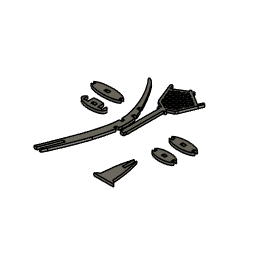
burnathome_model (Autodesk Fusion 360 design; units mm, degrees)
Autodesk Fusion 360 part; units mm, degrees
note: some values were not read from the file. Set by a fixed rule: which sketch regions a step uses.
(part 1 of 2)
sketch "Sketch1" plane through (0, 0, 0) normal (0, 0, 1) x (1, 0, 0)
  spline S0 degree 3 poles (105.7444, 14.5032) (117.4288, 44.6604) (130.3665, 74.6483) (136.8117, 106.4812) knots 0 0 0 0 1 1 1 1
  spline S1 degree 3 poles (135.284, 152.6044) (128.6212, 175.9715) (117.3015, 198.1451) (101.7627, 216.8286) knots 0 0 0 0 1 1 1 1
  spline S2 degree 3 poles (101.7627, 216.8286) (100.2225, 218.6487) (96.6852, 221.8312) (97.531, 222.5321) knots 0 0 0 0 1 1 1 1
  spline S3 degree 3 poles (97.531, 222.5321) (99.4549, 223.9712) (106.4176, 220.3297) (113.8276, 209.9742) knots 0 0 0 0 1 1 1 1
  spline S4 degree 3 poles (113.8276, 209.9742) (127.6672, 190.7251) (139.1986, 169.8205) (148.7703, 148.1491) knots 0 0 0 0 1 1 1 1
  spline S5 degree 3 poles (148.7593, 148.174) (152.834, 138.1049) (152.7256, 126.9178) (152.0453, 116.2604) knots 0 0 0 0 1 1 1 1
  spline S6 degree 3 poles (152.047, 116.2872) (150.3094, 104.2979) (146.4472, 89.1288) (141.1137, 70.5518) knots 0 0 0 0 1 1 1 1
  spline S7 degree 2 poles (161.9789, 170.2352) (154.8849, 179.5494) (137.874, 203.6318) knots 0 0 0 1 1 1
  spline S8 degree 3 poles (137.874, 203.6318) (145.0675, 206.7636) (154.3879, 210.8154) (161.9789, 214.1758) knots 0 0 0 0 1 1 1 1
  spline S9 degree 3 poles (161.9789, 214.1758) (170.0804, 210.3083) (178.4147, 206.771) (186.3736, 202.7014) knots 0 0 0 0 1 1 1 1
  spline S10 degree 3 poles (186.3736, 202.7014) (182.615, 197.9373) (162.2857, 169.7391) (161.9789, 170.2352) knots 0 0 0 0 1 1 1 1
  line L0 (161.9789, 214.1758) -> (161.9789, 165.1) construction
  line L1 (101.7627, 216.8286) -> (100.2225, 218.6487) construction
  line L2 (100.2225, 218.6487) -> (96.6852, 221.8312) construction
  line L3 (96.6852, 221.8312) -> (97.531, 222.5321) construction
  line L4 (97.531, 222.5321) -> (99.4549, 223.9712) construction
  line L5 (99.4549, 223.9712) -> (106.4176, 220.3297) construction
  line L6 (106.4176, 220.3297) -> (113.8276, 209.9742) construction
  line L7 (152.047, 116.2872) -> (150.3094, 104.2979) construction
  line L8 (150.3094, 104.2979) -> (146.4472, 89.1288) construction
  line L9 (146.4472, 89.1288) -> (141.1137, 70.5518) construction
  line L10 (119.1614, 37.5643) -> (123.5466, 35.8761)
  line L11 (123.5466, 35.8761) -> (109.8583, 0.3199)
  line L12 (119.1614, 37.5643) -> (104.7977, 0.254)
  spline S11 degree 3 poles (141.1137, 70.5518) (136.0968, 54.3686) (125.6817, 28.5289) (117.0593, 8.6966) knots 0 0 0 0 0.937383 0.937383 0.937383 0.937383
  line L13 (141.1137, 70.5518) -> (136.0968, 54.3686) construction
  line L14 (136.0968, 54.3686) -> (125.6817, 28.5289) construction
  line L15 (125.6817, 28.5289) -> (117.0593, 8.6966) construction
  spline S12 degree 3 poles (99.568, 0.254) (99.8499, 0.2503) (102.6483, 6.336) (105.7444, 14.5032) knots 0.351989 0.351989 0.351989 0.351989 1 1 1 1
  line L16 (99.568, 0.254) -> (99.8499, 0.2503) construction
  line L17 (99.8499, 0.2503) -> (102.6483, 6.336) construction
  line L18 (102.6483, 6.336) -> (105.7444, 14.5032) construction
  line L19 (202.385, 12.1082) -> (221.4351, 12.1082)
  line L20 (221.4351, 12.1082) -> (221.4351, 36.9579) construction
  line L21 (219.0856, 50.2082) -> (219.0856, 73.0762)
  line L22 (219.0856, 50.2082) -> (221.4351, 50.2082)
  arc A0 (209.8206, 17.9721) -> (202.385, 12.1082) centre (221.435, -4.4018) ccw
  spline S13 degree 5 poles (219.0856, 73.0762) (218.798, 72.0356) (218.2295, 69.9495) (217.3962, 66.8053) (216.327, 62.5819) (215.0787, 57.2456) (213.9414, 51.8447) (212.9362, 46.3723) (212.0737, 40.825) (211.3458, 35.2064) (210.736, 29.5227) (210.3279, 24.9291) (210.0601, 21.4598) (209.8977, 19.1364) (209.8206, 17.9721) knots 0 0 0 0 0 0 0.1 0.2 0.3 0.4 0.5 0.6 0.7 0.8 0.9 1 1 1 1 1 1
  line L23 (240.4851, 12.1082) -> (221.4351, 12.1082)
  arc A1 (240.4851, 12.1082) -> (233.0495, 17.9721) centre (221.4351, -4.4018) ccw
  line L24 (223.7846, 50.2082) -> (223.7846, 73.0762)
  spline S14 degree 5 poles (223.7846, 73.0762) (224.0721, 72.0356) (224.6406, 69.9495) (225.4739, 66.8053) (226.5431, 62.5819) (227.7914, 57.2456) (228.9287, 51.8447) (229.9339, 46.3723) (230.7964, 40.825) (231.5243, 35.2064) (232.1341, 29.5227) (232.5422, 24.9291) (232.81, 21.4598) (232.9724, 19.1364) (233.0495, 17.9721) knots 0 0 0 0 0 0 0.1 0.2 0.3 0.4 0.5 0.6 0.7 0.8 0.9 1 1 1 1 1 1
  line L25 (220.5921, 78.5288) -> (217.579, 67.6235)
  line L26 (210.2086, 23.8294) -> (209.4327, 12.1147)
  line L27 (222.278, 78.5288) -> (225.2911, 67.6235)
  line L28 (232.6616, 23.8294) -> (233.4374, 12.1147)
  line L29 (223.7846, 50.2082) -> (221.4351, 50.2082)
  line L30 (161.9789, 228.6) -> (161.9789, -25.4) construction
  line L31 (139.0297, 126.8561) -> (161.9789, 126.8561) construction
  line L32 (137.237, 162.3529) -> (161.9789, 162.3117) construction
  line L33 (143.7687, 145.0614) -> (161.9789, 145.0614) construction
  line L34 (156.4687, 142.7119) -> (143.7687, 142.7119)
  line L35 (143.7687, 142.7119) -> (143.7687, 147.4109)
  line L36 (143.7687, 147.4109) -> (156.4687, 147.4109)
  line L37 (156.4687, 147.4109) -> (156.4687, 142.7119)
  line L38 (156.4687, 142.7119) -> (143.7687, 147.4109) construction
  line L39 (143.7687, 142.7119) -> (156.4687, 147.4109) construction
  line L40 (161.9789, 108.9422) -> (146.0368, 108.9422) construction
  line L41 (155.5618, 111.2917) -> (146.0368, 111.2917)
  line L42 (146.0368, 111.2917) -> (146.0368, 106.5927)
  line L43 (146.0368, 106.5927) -> (155.5618, 106.5927)
  line L44 (155.5618, 106.5927) -> (155.5618, 111.2917)
  line L45 (155.5618, 111.2917) -> (146.0368, 106.5927) construction
  line L46 (146.0368, 111.2917) -> (155.5618, 106.5927) construction
  line L47 (147.0795, 159.9952) -> (137.237, 159.9952)
  line L48 (137.237, 159.9952) -> (137.237, 164.6942)
  line L49 (137.237, 164.6942) -> (147.0795, 164.6942)
  line L50 (147.0795, 164.6942) -> (147.0795, 159.9952)
  line L51 (147.0795, 159.9952) -> (137.237, 164.6942) construction
  line L52 (137.237, 159.9952) -> (147.0795, 164.6942) construction
  ellipse E0 centre (79.447, 160.9534) end of major axis (109.2158, 160.9534) minor radius 9.525
  line L53 (49.6782, 160.9534) -> (109.2158, 160.9534) construction
  line L54 (79.447, 151.4284) -> (79.447, 170.4784) construction
  line L55 (83.257, 158.6039) -> (75.637, 158.6039)
  line L56 (75.637, 158.6039) -> (75.637, 163.3029)
  line L57 (75.637, 163.3029) -> (83.257, 163.3029)
  line L58 (83.257, 163.3029) -> (83.257, 158.6039)
  line L59 (83.257, 158.6039) -> (75.637, 163.3029) construction
  line L60 (75.637, 158.6039) -> (83.257, 163.3029) construction
  line L61 (132.2063, 162.3613) -> (137.237, 162.3529) construction
  line L62 (137.1951, 145.0614) -> (143.7687, 145.0614) construction
  line L63 (146.0368, 108.9422) -> (137.3129, 108.9422) construction
  line L64 (54.6058, 163.3029) -> (44.7506, 163.3029)
  line L65 (44.7506, 163.3029) -> (44.7506, 158.6039)
  line L66 (44.7506, 158.6039) -> (54.6058, 158.6039)
  line L67 (54.6058, 158.6039) -> (54.6058, 163.3029)
  line L68 (54.6058, 163.3029) -> (44.7506, 158.6039) construction
  line L69 (44.7506, 163.3029) -> (54.6058, 158.6039) construction
  line L70 (104.2882, 158.6039) -> (114.1434, 158.6039)
  line L71 (114.1434, 158.6039) -> (114.1434, 163.3029)
  line L72 (114.1434, 163.3029) -> (104.2882, 163.3029)
  line L73 (104.2882, 163.3029) -> (104.2882, 158.6039)
  line L74 (104.2882, 158.6039) -> (114.1434, 163.3029) construction
  line L75 (114.1434, 158.6039) -> (104.2882, 163.3029) construction
  line L76 (237.743, 142.2845) -> (245.363, 146.9835) construction
  line L77 (259.7902, 146.9835) -> (259.7902, 142.2845)
  line L78 (274.1158, 142.2845) -> (274.1158, 146.9835)
  line L79 (208.9902, 146.9835) -> (223.3158, 142.2845) construction
  line L80 (208.9902, 146.9835) -> (208.9902, 142.2845)
  line L81 (223.3158, 142.2845) -> (223.3158, 146.9835)
  line L82 (259.7902, 142.2845) -> (274.1158, 142.2845)
  line L83 (245.363, 142.2845) -> (237.743, 142.2845)
  line L84 (245.363, 142.2845) -> (237.743, 146.9835) construction
  line L85 (259.7902, 142.2845) -> (274.1158, 146.9835) construction
  line L86 (237.743, 142.2845) -> (237.743, 146.9835)
  line L87 (208.9902, 142.2845) -> (223.3158, 142.2845)
  line L88 (245.363, 146.9835) -> (245.363, 142.2845)
  line L89 (274.1158, 142.2845) -> (259.7902, 146.9835) construction
  line L90 (274.1158, 146.9835) -> (259.7902, 146.9835)
  line L91 (223.3158, 146.9835) -> (208.9902, 146.9835)
  line L92 (237.743, 146.9835) -> (245.363, 146.9835)
  line L93 (223.3158, 146.9835) -> (208.9902, 142.2845) construction
  ellipse E1 centre (241.553, 144.634) end of major axis (266.953, 144.634) minor radius 9.525
  line L94 (216.153, 144.634) -> (266.953, 144.634) construction
  line L95 (241.553, 135.109) -> (241.553, 154.159) construction
  line L96 (91.1889, 125.3656) -> (83.5689, 125.3656)
  line L97 (91.1889, 125.3656) -> (83.5689, 130.0646) construction
  line L98 (83.5689, 130.0646) -> (91.1889, 130.0646)
  line L99 (83.5689, 125.3656) -> (83.5689, 130.0646)
  line L100 (91.1889, 130.0646) -> (91.1889, 125.3656)
  line L101 (83.5689, 125.3656) -> (91.1889, 130.0646) construction
  line L102 (225.1114, 106.1159) -> (225.1114, 110.8149)
  line L103 (268.2914, 106.1159) -> (257.1662, 110.8149) construction
  line L104 (213.9862, 110.8149) -> (225.1114, 106.1159) construction
  line L105 (257.1662, 106.1159) -> (268.2914, 110.8149) construction
  line L106 (244.3138, 106.1159) -> (237.9638, 106.1159)
  line L107 (257.1662, 106.1159) -> (268.2914, 106.1159)
  line L108 (225.1114, 110.8149) -> (213.9862, 110.8149)
  line L109 (244.3138, 106.1159) -> (237.9638, 110.8149) construction
  line L110 (257.1662, 110.8149) -> (257.1662, 106.1159)
  line L111 (213.9862, 110.8149) -> (213.9862, 106.1159)
  line L112 (225.1114, 110.8149) -> (213.9862, 106.1159) construction
  line L113 (213.9862, 106.1159) -> (225.1114, 106.1159)
  line L114 (268.2914, 110.8149) -> (257.1662, 110.8149)
  line L115 (237.9638, 110.8149) -> (244.3138, 110.8149)
  line L116 (237.9638, 106.1159) -> (237.9638, 110.8149)
  line L117 (244.3138, 110.8149) -> (244.3138, 106.1159)
  line L118 (237.9638, 106.1159) -> (244.3138, 110.8149) construction
  ellipse E2 centre (241.1388, 108.4654) end of major axis (262.7288, 108.4654) minor radius 9.525
  line L119 (219.5488, 108.4654) -> (262.7288, 108.4654) construction
  line L120 (241.1388, 98.9404) -> (241.1388, 117.9904) construction
  line L121 (268.2914, 106.1159) -> (268.2914, 110.8149)
  line L122 (158.1689, 176.53) -> (165.7889, 176.53)
  line L123 (165.7889, 176.53) -> (165.7889, 111.4565)
  line L124 (158.1689, 111.4565) -> (158.1689, 176.53)
  spline S15 degree 3 poles (161.8759, 205.8008) (166.2261, 203.7742) (170.5456, 201.8424) (174.7461, 199.881) knots 0.127739 0.127739 0.127739 0.127739 0.652669 0.652669 0.652669 0.652669
  spline S16 degree 3 poles (174.7461, 199.881) (172.3216, 196.5944) (169.4721, 192.7118) (166.7324, 188.9957) (165.1268, 186.8178) (163.5593, 184.6977) (162.1432, 182.7963) knots 0.254809 0.254809 0.254809 0.254809 0.50048 0.50048 0.50048 0.64446 0.64446 0.64446 0.64446
  spline S17 degree 3 poles (162.1432, 182.7963) (159.0509, 187.0323) (155.2878, 192.2652) (150.8627, 198.484) (150.4183, 199.1085) (149.9672, 199.743) (149.5094, 200.3875) knots 0.340954 0.340954 0.340954 0.340954 0.787557 0.787557 0.787557 0.83241 0.83241 0.83241 0.83241
  spline S18 degree 3 poles (149.5094, 200.3875) (153.6089, 202.1746) (157.8877, 204.0444) (161.8759, 205.8008) knots 0.36706 0.36706 0.36706 0.36706 0.864387 0.864387 0.864387 0.864387
  spline S19 degree 3 poles (136.8117, 106.4811) (136.8741, 106.7796) (136.9365, 107.0782) (136.999, 107.3768) (140.1243, 122.3208) (139.7101, 137.9614) (135.2839, 152.6046) knots 0 0 0 0 0.091508 0.091508 0.091508 1.091508 1.091508 1.091508 1.091508
  line L125 (144.1097, 129.2056) -> (133.9497, 129.2056)
  line L126 (133.9497, 129.2056) -> (133.9497, 124.5066)
  line L127 (133.9497, 124.5066) -> (144.1097, 124.5066)
  line L128 (144.1097, 124.5066) -> (144.1097, 129.2056)
  line L129 (144.1097, 129.2056) -> (133.9497, 124.5066) construction
  line L130 (133.9497, 129.2056) -> (144.1097, 124.5066) construction
  line L131 (69.3814, 125.4267) -> (77.7634, 125.4267)
  line L132 (77.7634, 125.4267) -> (77.7634, 136.487)
  line L133 (69.3814, 133.6454) -> (69.3814, 125.4267)
  line L134 (96.7076, 125.4267) -> (105.0896, 125.4267)
  line L135 (105.0896, 125.4267) -> (105.0896, 133.7524)
  line L136 (96.7076, 136.5214) -> (96.7076, 125.4267)
  ellipse E3 centre (87.3789, 127.7151) end of major axis (110.3281, 127.6837) minor radius 9.525 (69.3814, 133.6454) -> (105.0896, 133.7524) ccw
  ellipse E4 centre (87.3789, 127.7151) end of major axis (110.2537, 127.6848) minor radius 9.6559 (96.7076, 136.5214) -> (77.7634, 136.487) ccw
  line L137 (104.7977, 0.254) -> (99.568, 0.254)
  line L138 (158.8039, 111.4565) -> (158.8039, 106.68)
  line L139 (158.8039, 106.68) -> (165.1539, 106.68)
  line L140 (165.1539, 106.68) -> (165.1539, 111.4565)
  line L141 (165.7889, 111.4565) -> (165.1539, 111.4565)
  line L142 (158.8039, 111.4565) -> (158.1689, 111.4565)
  line L143 (109.8583, 0.3199) -> (113.0859, 0.3199)
  line L144 (117.0593, 8.6966) -> (113.0859, 0.3199)
  point P0 (213.0605, 46.8735)
  point P1 (229.8096, 46.8735)
  point P2 (152.4027, 126.8561)
  point P3 (150.1187, 145.0614)
  point P4 (142.1582, 162.3447)
  point P5 (150.7993, 108.9422)
  point P6 (142.1582, 162.3447)
  point P7 (79.447, 160.9534)
  point P8 (49.6782, 160.9534)
  point P9 (109.2158, 160.9534)
  point P10 (241.553, 144.634)
  point P11 (216.153, 144.634)
  point P12 (266.953, 144.634)
  point P13 (87.3789, 127.7151)
  point P14 (64.2667, 127.9032)
  point P15 (110.1696, 127.9032)
  point P16 (241.1388, 108.4654)
  point P17 (219.5488, 108.4654)
  point P18 (262.7288, 108.4654)
  point P19 (161.9789, 176.53)
  point P20 (140.3889, 108.9503)
  point P21 (136.5789, 145.0601)
  point P22 (139.0297, 126.8561)
  point P23 (69.3467, 127.9032)
  dimension "d2" = 4.699
  dimension "d4" = 38.1
  dimension "d6" = 2.3495
  dimension "d9" = 38.1
  dimension "d12" = 12.7
  dimension "d13" = 4.699
  dimension "d16" = 9.525
  dimension "d17" = 4.699
  dimension "d18" = 9.8425
  dimension "d19" = 4.699
  dimension "d20" = 59.5376
  dimension "d21" = 19.05
  dimension "d22" = 7.62
  dimension "d23" = 4.699
  dimension "d24" = 9.8552
  dimension "d25" = 4.699
  dimension "d26" = 9.8552
  dimension "d27" = 4.699
  dimension "d28" = 50.8
  dimension "d29" = 19.05
  dimension "d30" = 7.62
  dimension "d31" = 4.699
  dimension "d32" = 14.3256
  dimension "d33" = 4.699
  dimension "d34" = 14.3256
  dimension "d35" = 4.699
  dimension "d36" = 45.8984
  dimension "d37" = 19.05
  dimension "d38" = 7.62
  dimension "d39" = 4.699
  dimension "d44" = 43.18
  dimension "d45" = 19.05
  dimension "d46" = 6.35
  dimension "d47" = 4.699
  dimension "d48" = 11.1252
  dimension "d49" = 4.699
  dimension "d50" = 11.1252
  dimension "d51" = 4.699
  dimension "d52" = 7.62
  dimension "d54" = 7.62
  dimension "d61" = 21.59
  dimension "d63" = 25.4
  dimension "d64" = 29.7726
  dimension "d65" = 22.9492
  dimension "d66" = 10.16
  dimension "d67" = 4.699
  dimension "d68" = 5.08
  dimension "d70" = 8.382
  dimension "d71" = 8.382
  dimension "d72" = 5.08
  dimension "d74" = 6.35
  constraint vertical L0
  constraint coincident S7.start L0
  constraint perpendicular L10 L12
  constraint perpendicular L10 L11
  constraint horizontal L19
  constraint perpendicular L19 L20
  constraint perpendicular L19 L21
  constraint coincident L20 L22.end
  constraint midpoint L21.end L25
  constraint midpoint A0.start L26
  constraint symmetric L19.start L20 L23.start
  constraint symmetric L19.end L20 L23.end
  constraint symmetric L20 L21.end L24.end
  constraint symmetric L20 L21.start L24.start
  constraint symmetric L20 A0 A1
  constraint symmetric L20 P0 P1
  constraint symmetric L20 A0.start A1.end
  constraint symmetric L20 L22.end L29.end
  constraint symmetric L20 L25.start L27.start
  constraint symmetric L20 L25.end L27.end
  constraint symmetric L20 L26.start L28.start
  constraint symmetric L20 L26.end L28.end
  constraint vertical L30
  constraint coincident L30 L31.end
  constraint perpendicular L30 L31
  constraint coincident S8.end L30
  constraint coincident L0 L32.end
  constraint coincident L30 L33.end
  constraint perpendicular L30 L33
  constraint coincident L31 P2
  constraint coincident S5 P2
  constraint horizontal L34
  constraint perpendicular L34 L35
  constraint parallel L34 L36
  constraint parallel L35 L37
  constraint coincident L38 P3
  constraint coincident L39 P3
  constraint coincident L33 P3
  constraint coincident S4 P3
  constraint coincident L32 P6
  constraint coincident S4 P6
  constraint coincident L30 L40.start
  constraint perpendicular L30 L40
  constraint horizontal L41
  constraint perpendicular L41 L42
  constraint parallel L41 L43
  constraint parallel L42 L44
  constraint coincident L45 P5
  constraint coincident L46 P5
  constraint coincident S6 P5
  constraint coincident L40 P5
  constraint horizontal L47
  constraint perpendicular L47 L48
  constraint parallel L47 L49
  constraint parallel L48 L50
  constraint coincident L51 P6
  constraint coincident L52 P6
  constraint coincident P6 P4
  constraint coincident S1 L61.start
  constraint coincident L62.start S19
  constraint coincident L63.end S19
  constraint horizontal L53
  constraint coincident E0 P8
  constraint coincident E0 P9
  constraint coincident E0 L54.start
  constraint coincident E0 L54.end
  constraint horizontal L55
  constraint perpendicular L55 L56
  constraint parallel L55 L57
  constraint parallel L56 L58
  constraint coincident L59 P7
  constraint coincident L60 P7
  constraint coincident P7 E0.centre
  constraint coincident L48 L32.start
  constraint coincident P6 L61
  constraint coincident L35 L33.start
  constraint perpendicular L30 L62
  constraint coincident L42 L40.end
  constraint perpendicular L30 L63
  constraint horizontal L64
  constraint perpendicular L64 L65
  constraint parallel L64 L66
  constraint parallel L65 L67
  constraint coincident L68 P8
  constraint coincident L69 P8
  constraint coincident P8 L53.start
  constraint horizontal L70
  constraint perpendicular L70 L71
  constraint parallel L70 L72
  constraint parallel L71 L73
  constraint coincident L74 P9
  constraint coincident L75 P9
  constraint coincident P9 L53.end
  constraint horizontal L94
  constraint coincident P11 E1
  constraint coincident P12 E1
  constraint coincident L95.start E1
  constraint coincident L95.end E1
  constraint horizontal L83
  constraint perpendicular L83 L86
  constraint parallel L83 L92
  constraint parallel L86 L88
  constraint coincident P10 L84
  constraint coincident P10 L76
  constraint coincident P10 E1.centre
  constraint horizontal L91
  constraint perpendicular L80 L91
  constraint parallel L87 L91
  constraint parallel L80 L81
  constraint coincident P11 L93
  constraint coincident P11 L79
  constraint coincident P11 L94.start
  constraint horizontal L82
  constraint perpendicular L78 L82
  constraint parallel L82 L90
  constraint parallel L77 L78
  constraint coincident P12 L85
  constraint coincident P12 L89
  constraint coincident P12 L94.end
  constraint horizontal L96
  constraint perpendicular L96 L99
  constraint parallel L96 L98
  constraint parallel L99 L100
  constraint coincident P13 L97
  constraint coincident P13 L101
  constraint coincident P13 E3.centre
  constraint horizontal L119
  constraint coincident P17 E2
  constraint coincident P18 E2
  constraint coincident L120.start E2
  constraint coincident L120.end E2
  constraint horizontal L106
  constraint perpendicular L106 L116
  constraint parallel L106 L115
  constraint parallel L116 L117
  constraint coincident P16 L109
  constraint coincident P16 L118
  constraint coincident P16 E2.centre
  constraint horizontal L108
  constraint perpendicular L108 L111
  constraint parallel L108 L113
  constraint parallel L102 L111
  constraint coincident P17 L112
  constraint coincident P17 L104
  constraint coincident P17 L119.start
  constraint horizontal L107
  constraint perpendicular L107 L121
  constraint parallel L107 L114
  constraint parallel L110 L121
  constraint coincident P18 L105
  constraint coincident P18 L103
  constraint coincident P18 L119.end
  constraint horizontal L122
  constraint vertical L123
  constraint horizontal L141
  constraint vertical L124
  constraint midpoint L122 P19
  constraint coincident L30 P19
  constraint coincident S19 P22
  constraint horizontal L125
  constraint perpendicular L125 L126
  constraint parallel L125 L127
  constraint parallel L126 L128
  constraint coincident L129 P22
  constraint coincident L130 P22
  constraint coincident P22 L31.start
  constraint horizontal L131
  constraint vertical L132
  constraint vertical L133
  constraint horizontal L134
  constraint vertical L135
  constraint vertical L136
  constraint concentric E3 E4
  constraint horizontal L137
  constraint coincident S12.start L16.start
  constraint coincident L138.start L141
  constraint perpendicular L138 L141
  constraint perpendicular L138 L139
  constraint perpendicular L140 L141
  constraint collinear L141 L142
  constraint equal L141 L142
  constraint horizontal L143
  measures "d2" distance of L10.start L10.end
  measures "d4" distance of L10.end L11.end
  measures "d6" distance of L20 L21
  measures "d9" distance of L19 L22
  measures "d12" distance of L35.end L36.end
  measures "d13" distance of L34.end L35.end
  measures "d16" distance of L42.end L43.end
  measures "d17" distance of L41.end L42.end
  measures "d18" distance of L48.end L49.end
  measures "d19" distance of L47.end L48.end
  measures "d20" distance of E0
  measures "d22" distance of L56.end L57.end
  measures "d23" distance of L55.end L56.end
  measures "d24" distance of L65.end L66.end
  measures "d25" distance of L64.end L65.end
  measures "d26" distance of L71.end L72.end
  measures "d27" distance of L70.end L71.end
  measures "d28" distance of E1
  measures "d30" distance of L84.end L76.end
  measures "d31" distance of L84.end L76.start
  measures "d32" distance of L79.end L80.end
  measures "d33" distance of L79.start L80.end
  measures "d34" distance of L78.end L77.start
  measures "d35" distance of L78.start L78.end
  measures "d36" distance of E3
  measures "d38" distance of L97.end L98.end
  measures "d39" distance of L97.end L96.end
  measures "d44" distance of E2
  measures "d46" distance of L109.end L115.end
  measures "d47" distance of L109.end L106.end
  measures "d48" distance of L102.start L111.end
  measures "d49" distance of L104.start L111.end
  measures "d50" distance of L105.end L103.end
  measures "d51" distance of L103.start L105.end
  measures "d52" distance of L122.start L122.end
  measures "d61" distance of L40.start P20
  measures "d63" distance of L33.end P21
  measures "d64" horizontal distance of L32.end L61.start
  measures "d65" distance of L31.end P22
  measures "d66" distance of L126.end L127.end
  measures "d67" distance of L125.end L126.end
  measures "d68" distance of P14 P23
  measures "d70" distance of L131.start L131.end
  measures "d71" distance of L134.start L134.end
  measures "d72" distance of P15 L135
  measures "d74" distance of L138.end L139.end
extrude "Extrude2" add sketch "Sketch1" along normal blind 4.699 contours S0 S1 S2 S3 S4 S5 S6 L10 L11 L12 S11 S12 L34 L35 L36 L41 L42 L43 L47 L48 L49 S19 L125 L127 L128 L137 L143 L144 | S7 S10 L123 L124 L138 L139 L140 L141 L142 | S7 S10 L122 L123 L124 | S7 S8 S9 S10 L122 L123 L124 | L19 L21 L22 A0 S13 L23 A1 L24 S14 L29 | E0 L64 L66 L67 L70 L72 L73 | L77 L81 L82 L87 L90 L91 E1 | L102 L107 L108 L110 L113 L114 E2 | L131 L132 L133 L134 L135 L136 E3 E4 makes body 1 at (252.4331, 149.0861, 0) makes body 2 at (79.6986, 130.6594, 0) makes body 3 at (175.6362, 192.5122, 0) makes body 4 at (251.5125, 112.6791, 0) makes body 5 at (70.1789, 161.7848, 0) makes body 6 at (221.4351, 26.658, 0) makes body 7 at (133.7227, 78.9656, 0)
sketch "Sketch2" plane through (0, 0, 4.699) normal (0, 0, 1) x (-1, 0, 0)
  line L0 (-158.8039, -106.68) -> (-165.1539, -106.68)
  line L1 (-165.1539, -106.68) -> (-165.1539, -111.4565)
  line L2 (-165.1539, -111.4565) -> (-165.7889, -111.4565)
  line L3 (-165.7889, -111.4565) -> (-165.7889, -174.9541)
  line L4 (-158.1689, -175.331) -> (-158.1689, -111.4565)
  line L5 (-158.1689, -111.4565) -> (-158.8039, -111.4565)
  line L6 (-158.8039, -111.4565) -> (-158.8039, -106.68)
  line L7 (-168.7102, -180.8892) -> (-170.2391, -183.9833)
  line L8 (-191.2572, -223.0614) -> (-194.8572, -232.3981)
  line L9 (-191.7134, -233.6497) -> (-188.2271, -224.8966)
  line L10 (-134.3845, -219.435) -> (-143.8837, -195.7123)
  line L11 (-165.9602, -186.0971) -> (-178.2439, -192.1658)
  line L12 (-188.2271, -224.8966) -> (-165.345, -239.08)
  line L13 (-165.2823, -243.1079) -> (-162.0641, -241.1134)
  line L14 (-157.0243, -240.1702) -> (-158.7831, -239.08)
  line L15 (-153.8892, -183.9833) -> (-155.4181, -180.8892)
  line L16 (-129.2709, -232.3981) -> (-132.8709, -223.0612)
  line L17 (-170.2391, -183.9833) -> (-165.9602, -186.0971)
  line L18 (-162.0641, -241.1134) -> (-158.8458, -243.1079)
  line L19 (-194.8572, -232.3981) -> (-191.7134, -233.6497)
  line L20 (-145.8842, -192.1658) -> (-158.1682, -186.0971)
  line L21 (-135.9013, -224.8966) -> (-132.4147, -233.6497)
  line L22 (-165.345, -239.08) -> (-167.1041, -240.1702)
  line L23 (-165.7889, -182.3323) -> (-168.7102, -180.8892)
  line L24 (-180.2447, -195.7123) -> (-189.7436, -219.435)
  line L25 (-132.4147, -233.6497) -> (-129.2709, -232.3981)
  line L26 (-155.4181, -180.8892) -> (-158.1689, -182.2481)
  line L27 (-158.8458, -243.1079) -> (-157.0243, -240.1702)
  line L28 (-158.1682, -186.0971) -> (-153.8892, -183.9833)
  line L29 (-158.7831, -239.08) -> (-135.9013, -224.8966)
  line L30 (-167.1041, -240.1702) -> (-165.2823, -243.1079)
  line L31 (-150.8628, -193.556) -> (-150.8628, -195.1061)
  line L32 (-150.8628, -195.1061) -> (-147.768, -195.1061)
  line L33 (-147.768, -195.1061) -> (-147.7791, -195.0794)
  line L34 (-147.7791, -195.0794) -> (-150.8628, -193.556)
  line L35 (-152.1466, -192.9219) -> (-157.4944, -190.2798)
  line L36 (-152.1466, -195.1061) -> (-152.1466, -192.9219)
  line L37 (-157.4944, -190.2798) -> (-157.4944, -195.1061)
  line L38 (-157.4944, -195.1061) -> (-152.1466, -195.1061)
  line L39 (-161.8363, -188.1347) -> (-164.116, -189.2274)
  line L40 (-164.116, -195.1061) -> (-158.7509, -195.1061)
  line L41 (-158.7509, -189.6587) -> (-161.8363, -188.1347)
  line L42 (-164.116, -189.2274) -> (-164.116, -195.1061)
  line L43 (-158.7509, -195.1061) -> (-158.7509, -189.6587)
  line L44 (-165.3649, -195.1061) -> (-165.3649, -189.8259)
  line L45 (-170.8485, -192.4544) -> (-170.8485, -195.1061)
  line L46 (-170.8485, -195.1061) -> (-165.3649, -195.1061)
  line L47 (-165.3649, -189.8259) -> (-170.8485, -192.4544)
  line L48 (-172.1153, -195.1061) -> (-172.1153, -193.0618)
  line L49 (-176.3048, -195.07) -> (-176.3191, -195.1061)
  line L50 (-172.1153, -193.0618) -> (-176.3048, -195.07)
  line L51 (-176.3191, -195.1061) -> (-172.1153, -195.1061)
  line L52 (-145.6673, -201.6101) -> (-145.6673, -200.3815)
  line L53 (-150.8628, -196.4098) -> (-150.8628, -201.6101)
  line L54 (-150.8628, -201.6101) -> (-145.6673, -201.6101)
  line L55 (-145.6673, -200.3815) -> (-147.2493, -196.4098)
  line L56 (-147.2493, -196.4098) -> (-150.8628, -196.4098)
  line L57 (-152.1466, -196.4098) -> (-157.4944, -196.4098)
  line L58 (-157.4944, -201.6101) -> (-152.1466, -201.6101)
  line L59 (-157.4944, -196.4098) -> (-157.4944, -201.6101)
  line L60 (-152.1466, -201.6101) -> (-152.1466, -196.4098)
  line L61 (-158.7509, -201.6101) -> (-158.7509, -196.4098)
  line L62 (-158.7509, -196.4098) -> (-164.116, -196.4098)
  line L63 (-164.116, -201.6101) -> (-158.7509, -201.6101)
  line L64 (-164.116, -196.4098) -> (-164.116, -201.6101)
  line L65 (-165.3649, -201.6101) -> (-165.3649, -196.4098)
  line L66 (-170.8485, -196.4098) -> (-170.8485, -201.6101)
  line L67 (-165.3649, -196.4098) -> (-170.8485, -196.4098)
  line L68 (-170.8485, -201.6101) -> (-165.3649, -201.6101)
  line L69 (-172.1153, -196.4098) -> (-176.8407, -196.4098)
  line L70 (-178.9203, -201.6101) -> (-172.1153, -201.6101)
  line L71 (-176.8407, -196.4098) -> (-178.9203, -201.6101)
  line L72 (-172.1153, -201.6101) -> (-172.1153, -196.4098)
  line L73 (-142.5384, -208.2364) -> (-144.3532, -203.6796)
  line L74 (-144.3532, -208.2364) -> (-142.5384, -208.2364)
  line L75 (-144.3532, -203.6796) -> (-144.3532, -208.2364)
  line L76 (-150.8628, -202.894) -> (-150.8628, -208.2364)
  line L77 (-145.6673, -202.894) -> (-150.8628, -202.894)
  line L78 (-150.8628, -208.2364) -> (-145.6673, -208.2364)
  line L79 (-145.6673, -208.2364) -> (-145.6673, -202.894)
  line L80 (-152.1466, -202.894) -> (-157.4944, -202.894)
  line L81 (-157.4944, -202.894) -> (-157.4944, -208.2364)
  line L82 (-157.4944, -208.2364) -> (-152.1466, -208.2364)
  line L83 (-152.1466, -208.2364) -> (-152.1466, -202.894)
  line L84 (-158.7509, -208.2364) -> (-158.7509, -202.894)
  line L85 (-164.116, -208.2364) -> (-158.7509, -208.2364)
  line L86 (-158.7509, -202.894) -> (-164.116, -202.894)
  line L87 (-164.116, -202.894) -> (-164.116, -208.2364)
  line L88 (-170.8485, -208.2364) -> (-165.3649, -208.2364)
  line L89 (-165.3649, -208.2364) -> (-165.3649, -202.894)
  line L90 (-170.8485, -202.894) -> (-170.8485, -208.2364)
  line L91 (-165.3649, -202.894) -> (-170.8485, -202.894)
  line L92 (-179.175, -208.2364) -> (-172.1153, -208.2364)
  line L93 (-172.1153, -208.2364) -> (-172.1153, -202.894)
  line L94 (-172.1153, -202.894) -> (-179.175, -202.894)
  line L95 (-179.175, -202.894) -> (-179.175, -208.2364)
  line L96 (-181.031, -208.2364) -> (-180.9883, -208.2364)
  line L97 (-142.0333, -209.5039) -> (-144.3532, -209.5039)
  line L98 (-139.8995, -214.8606) -> (-142.0333, -209.5039)
  line L99 (-144.3532, -209.5039) -> (-144.3532, -214.8606)
  line L100 (-144.3532, -214.8606) -> (-139.8995, -214.8606)
  line L101 (-145.6673, -214.8606) -> (-145.6673, -209.5039)
  line L102 (-145.6673, -209.5039) -> (-150.8628, -209.5039)
  line L103 (-150.8628, -209.5039) -> (-150.8628, -214.8606)
  line L104 (-150.8628, -214.8606) -> (-145.6673, -214.8606)
  line L105 (-157.4944, -209.5039) -> (-157.4944, -214.8606)
  line L106 (-157.4944, -214.8606) -> (-152.1466, -214.8606)
  line L107 (-152.1466, -209.5039) -> (-157.4944, -209.5039)
  line L108 (-152.1466, -214.8606) -> (-152.1466, -209.5039)
  line L109 (-164.116, -209.5039) -> (-164.116, -214.8606)
  line L110 (-164.116, -214.8606) -> (-158.7509, -214.8606)
  line L111 (-158.7509, -214.8606) -> (-158.7509, -209.5039)
  line L112 (-158.7509, -209.5039) -> (-164.116, -209.5039)
  line L113 (-165.3649, -209.5039) -> (-170.8485, -209.5039)
  line L114 (-170.8485, -209.5039) -> (-170.8485, -214.8606)
  line L115 (-165.3649, -214.8606) -> (-165.3649, -209.5039)
  line L116 (-170.8485, -214.8606) -> (-165.3649, -214.8606)
  line L117 (-172.1153, -209.5039) -> (-179.175, -209.5039)
  line L118 (-172.1153, -214.8606) -> (-172.1153, -209.5039)
  line L119 (-179.175, -209.5039) -> (-179.175, -214.8606)
  line L120 (-179.175, -214.8606) -> (-172.1153, -214.8606)
  line L121 (-180.4883, -214.8606) -> (-180.4883, -209.5039)
  line L122 (-184.2184, -214.8606) -> (-180.4883, -214.8606)
  line L123 (-182.0764, -209.5039) -> (-184.2184, -214.8606)
  line L124 (-180.4883, -209.5039) -> (-182.0764, -209.5039)
  line L125 (-137.2111, -221.6104) -> (-139.4, -216.1156)
  line L126 (-139.4, -216.1156) -> (-144.3532, -216.1156)
  line L127 (-144.3532, -221.6104) -> (-137.2111, -221.6104)
  line L128 (-144.3532, -216.1156) -> (-144.3532, -221.6104)
  line L129 (-145.6673, -216.1156) -> (-150.8628, -216.1156)
  line L130 (-150.8628, -216.1156) -> (-150.8628, -221.6104)
  line L131 (-145.6673, -221.6104) -> (-145.6673, -216.1156)
  line L132 (-150.8628, -221.6104) -> (-145.6673, -221.6104)
  line L133 (-152.1466, -221.6104) -> (-152.1466, -216.1156)
  line L134 (-157.4944, -221.6104) -> (-152.1466, -221.6104)
  line L135 (-157.4944, -216.1156) -> (-157.4944, -221.6104)
  line L136 (-152.1466, -216.1156) -> (-157.4944, -216.1156)
  line L137 (-158.7509, -221.6104) -> (-158.7509, -216.1156)
  line L138 (-164.116, -221.6104) -> (-158.7509, -221.6104)
  line L139 (-158.7509, -216.1156) -> (-164.116, -216.1156)
  line L140 (-164.116, -216.1156) -> (-164.116, -221.6104)
  line L141 (-165.3649, -216.1156) -> (-170.8485, -216.1156)
  line L142 (-170.8485, -216.1156) -> (-170.8485, -221.6104)
  line L143 (-165.3649, -221.6104) -> (-165.3649, -216.1156)
  line L144 (-170.8485, -221.6104) -> (-165.3649, -221.6104)
  line L145 (-179.175, -216.1156) -> (-179.175, -221.6104)
  line L146 (-172.1153, -216.1156) -> (-179.175, -216.1156)
  line L147 (-179.175, -221.6104) -> (-172.1153, -221.6104)
  line L148 (-172.1153, -221.6104) -> (-172.1153, -216.1156)
  line L149 (-180.4883, -221.6104) -> (-180.4883, -216.1156)
  line L150 (-180.4883, -216.1156) -> (-184.7207, -216.1156)
  line L151 (-184.7207, -216.1156) -> (-186.9179, -221.6104)
  line L152 (-186.9179, -221.6104) -> (-180.4883, -221.6104)
  line L153 (-184.9329, -222.8483) -> (-180.4883, -225.5534)
  line L154 (-180.4883, -225.5534) -> (-180.4883, -222.8483)
  line L155 (-180.4883, -222.8483) -> (-184.9329, -222.8483)
  line L156 (-144.3532, -222.8483) -> (-144.3532, -226.0681)
  line L157 (-144.3532, -226.0681) -> (-139.1589, -222.8483)
  line L158 (-139.1589, -222.8483) -> (-144.3532, -222.8483)
  line L159 (-145.6673, -226.8822) -> (-145.6673, -222.8483)
  line L160 (-150.8628, -229.9223) -> (-150.5712, -229.9223)
  line L161 (-145.6673, -222.8483) -> (-150.8628, -222.8483)
  line L162 (-150.5712, -229.9223) -> (-145.6673, -226.8822)
  line L163 (-150.8628, -222.8483) -> (-150.8628, -229.9223)
  line L164 (-157.4944, -222.8483) -> (-157.4944, -229.9223)
  line L165 (-152.1466, -229.9223) -> (-152.1466, -222.8483)
  line L166 (-157.4944, -229.9223) -> (-152.1466, -229.9223)
  line L167 (-152.1466, -222.8483) -> (-157.4944, -222.8483)
  line L168 (-158.7509, -222.8483) -> (-164.116, -222.8483)
  line L169 (-164.116, -229.9223) -> (-158.7509, -229.9223)
  line L170 (-158.7509, -229.9223) -> (-158.7509, -222.8483)
  line L171 (-164.116, -222.8483) -> (-164.116, -229.9223)
  line L172 (-170.8485, -222.8483) -> (-170.8485, -229.9223)
  line L173 (-165.3649, -229.9223) -> (-165.3649, -222.8483)
  line L174 (-165.3649, -222.8483) -> (-170.8485, -222.8483)
  line L175 (-170.8485, -229.9223) -> (-165.3649, -229.9223)
  line L176 (-179.175, -226.3526) -> (-173.31, -229.9223)
  line L177 (-172.1153, -222.8483) -> (-179.175, -222.8483)
  line L178 (-173.31, -229.9223) -> (-172.1153, -229.9223)
  line L179 (-179.175, -222.8483) -> (-179.175, -226.3526)
  line L180 (-172.1153, -229.9223) -> (-172.1153, -222.8483)
  line L181 (-157.4944, -231.2356) -> (-157.4944, -234.2135)
  line L182 (-152.6899, -231.2356) -> (-157.4944, -231.2356)
  line L183 (-157.4944, -234.2135) -> (-152.6899, -231.2356)
  line L184 (-165.3649, -234.7576) -> (-165.3649, -231.2356)
  line L185 (-165.3649, -231.2356) -> (-170.8485, -231.2356)
  line L186 (-170.8485, -231.2356) -> (-170.8485, -231.4199)
  line L187 (-170.8485, -231.4199) -> (-165.3649, -234.7576)
  line L188 (-161.637, -236.7813) -> (-158.947, -235.114)
  line L189 (-163.8746, -231.4856) -> (-163.8746, -235.4192)
  line L190 (-158.947, -231.4856) -> (-163.8746, -231.4856)
  line L191 (-163.8746, -235.4192) -> (-161.637, -236.7813)
  line L192 (-158.947, -235.114) -> (-158.947, -231.4856)
  line L193 (-191.2572, -223.0614) -> (-180.2447, -195.7123)
  line L194 (-178.2439, -192.1658) -> (-180.2447, -195.7123)
  line L195 (-145.8842, -192.1658) -> (-143.8837, -195.7123)
  line L196 (-134.3845, -219.435) -> (-132.8709, -223.0612)
  line L197 (-158.1689, -175.331) -> (-158.1689, -182.2481)
  line L198 (-165.7889, -174.9541) -> (-165.7889, -182.3323)
  line L199 (-163.3746, -235.1382) -> (-161.6393, -236.1945)
  line L200 (-161.6393, -236.1945) -> (-159.447, -234.8356)
  line L201 (-159.447, -234.8356) -> (-159.447, -231.9856)
  line L202 (-159.447, -231.9856) -> (-163.3746, -231.9856)
  line L203 (-163.3746, -231.9856) -> (-163.3746, -235.1382)
  line L204 (-169.3681, -231.7356) -> (-165.8649, -233.8679)
  line L205 (-165.8649, -233.8679) -> (-165.8649, -231.7356)
  line L206 (-165.8649, -231.7356) -> (-169.3681, -231.7356)
  line L207 (-156.9944, -233.3153) -> (-154.4457, -231.7356)
  line L208 (-154.4457, -231.7356) -> (-156.9944, -231.7356)
  line L209 (-156.9944, -231.7356) -> (-156.9944, -233.3153)
  line L210 (-173.1698, -229.4223) -> (-172.6153, -229.4223)
  line L211 (-172.6153, -229.4223) -> (-172.6153, -223.3483)
  line L212 (-172.6153, -223.3483) -> (-178.675, -223.3483)
  line L213 (-178.675, -223.3483) -> (-178.675, -226.0716)
  line L214 (-178.675, -226.0716) -> (-173.1698, -229.4223)
  line L215 (-180.9883, -223.3483) -> (-183.1496, -223.3483)
  line L216 (-183.1496, -223.3483) -> (-180.9883, -224.6638)
  line L217 (-180.9883, -224.6638) -> (-180.9883, -223.3483)
  line L218 (-170.3485, -229.4223) -> (-165.8649, -229.4223)
  line L219 (-165.8649, -229.4223) -> (-165.8649, -223.3483)
  line L220 (-165.8649, -223.3483) -> (-170.3485, -223.3483)
  line L221 (-170.3485, -223.3483) -> (-170.3485, -229.4223)
  line L222 (-163.616, -229.4223) -> (-159.2509, -229.4223)
  line L223 (-159.2509, -229.4223) -> (-159.2509, -223.3483)
  line L224 (-159.2509, -223.3483) -> (-163.616, -223.3483)
  line L225 (-163.616, -223.3483) -> (-163.616, -229.4223)
  line L226 (-156.9944, -229.4223) -> (-152.6466, -229.4223)
  line L227 (-152.6466, -229.4223) -> (-152.6466, -223.3483)
  line L228 (-152.6466, -223.3483) -> (-156.9944, -223.3483)
  line L229 (-156.9944, -223.3483) -> (-156.9944, -229.4223)
  line L230 (-150.3628, -223.3483) -> (-150.3628, -229.2048)
  line L231 (-150.3628, -229.2048) -> (-146.1673, -226.6039)
  line L232 (-146.1673, -226.6039) -> (-146.1673, -223.3483)
  line L233 (-146.1673, -223.3483) -> (-150.3628, -223.3483)
  line L234 (-143.8532, -223.3483) -> (-143.8532, -225.1699)
  line L235 (-143.8532, -225.1699) -> (-140.9146, -223.3483)
  line L236 (-140.9146, -223.3483) -> (-143.8532, -223.3483)
  line L237 (-184.3821, -216.6156) -> (-186.1794, -221.1104)
  line L238 (-186.1794, -221.1104) -> (-180.9883, -221.1104)
  line L239 (-180.9883, -221.1104) -> (-180.9883, -216.6156)
  line L240 (-180.9883, -216.6156) -> (-184.3821, -216.6156)
  line L241 (-178.675, -216.6156) -> (-178.675, -221.1104)
  line L242 (-178.675, -221.1104) -> (-172.6153, -221.1104)
  line L243 (-172.6153, -221.1104) -> (-172.6153, -216.6156)
  line L244 (-172.6153, -216.6156) -> (-178.675, -216.6156)
  line L245 (-143.8532, -221.1104) -> (-137.9485, -221.1104)
  line L246 (-137.9485, -221.1104) -> (-139.739, -216.6156)
  line L247 (-139.739, -216.6156) -> (-143.8532, -216.6156)
  line L248 (-143.8532, -216.6156) -> (-143.8532, -221.1104)
  line L249 (-170.3485, -221.1104) -> (-165.8649, -221.1104)
  line L250 (-165.8649, -221.1104) -> (-165.8649, -216.6156)
  line L251 (-165.8649, -216.6156) -> (-170.3485, -216.6156)
  line L252 (-170.3485, -216.6156) -> (-170.3485, -221.1104)
  line L253 (-146.1673, -221.1104) -> (-146.1673, -216.6156)
  line L254 (-146.1673, -216.6156) -> (-150.3628, -216.6156)
  line L255 (-150.3628, -216.6156) -> (-150.3628, -221.1104)
  line L256 (-150.3628, -221.1104) -> (-146.1673, -221.1104)
  line L257 (-156.9944, -216.6156) -> (-156.9944, -221.1104)
  line L258 (-156.9944, -221.1104) -> (-152.6466, -221.1104)
  line L259 (-152.6466, -221.1104) -> (-152.6466, -216.6156)
  line L260 (-152.6466, -216.6156) -> (-156.9944, -216.6156)
  line L261 (-163.616, -216.6156) -> (-163.616, -221.1104)
  line L262 (-163.616, -221.1104) -> (-159.2509, -221.1104)
  line L263 (-159.2509, -221.1104) -> (-159.2509, -216.6156)
  line L264 (-159.2509, -216.6156) -> (-163.616, -216.6156)
  line L265 (-180.9883, -210.0039) -> (-181.7379, -210.0039)
  line L266 (-181.7379, -210.0039) -> (-183.4799, -214.3606)
  line L267 (-183.4799, -214.3606) -> (-180.9883, -214.3606)
  line L268 (-180.9883, -214.3606) -> (-180.9883, -210.0039)
  line L269 (-142.3724, -210.0039) -> (-143.8532, -210.0039)
  line L270 (-143.8532, -210.0039) -> (-143.8532, -214.3606)
  line L271 (-143.8532, -214.3606) -> (-140.6369, -214.3606)
  line L272 (-140.6369, -214.3606) -> (-142.3724, -210.0039)
  line L273 (-163.616, -214.3606) -> (-159.2509, -214.3606)
  line L274 (-159.2509, -214.3606) -> (-159.2509, -210.0039)
  line L275 (-159.2509, -210.0039) -> (-163.616, -210.0039)
  line L276 (-163.616, -210.0039) -> (-163.616, -214.3606)
  line L277 (-152.6466, -210.0039) -> (-156.9944, -210.0039)
  line L278 (-156.9944, -210.0039) -> (-156.9944, -214.3606)
  line L279 (-156.9944, -214.3606) -> (-152.6466, -214.3606)
  line L280 (-152.6466, -214.3606) -> (-152.6466, -210.0039)
  line L281 (-146.1673, -210.0039) -> (-150.3628, -210.0039)
  line L282 (-150.3628, -210.0039) -> (-150.3628, -214.3606)
  line L283 (-150.3628, -214.3606) -> (-146.1673, -214.3606)
  line L284 (-146.1673, -214.3606) -> (-146.1673, -210.0039)
  line L285 (-170.3485, -210.0039) -> (-170.3485, -214.3606)
  line L286 (-170.3485, -214.3606) -> (-165.8649, -214.3606)
  line L287 (-165.8649, -214.3606) -> (-165.8649, -210.0039)
  line L288 (-165.8649, -210.0039) -> (-170.3485, -210.0039)
  line L289 (-172.6153, -210.0039) -> (-178.675, -210.0039)
  line L290 (-178.675, -210.0039) -> (-178.675, -214.3606)
  line L291 (-178.675, -214.3606) -> (-172.6153, -214.3606)
  line L292 (-172.6153, -214.3606) -> (-172.6153, -210.0039)
  line L293 (-143.2758, -207.7364) -> (-143.8532, -206.2865)
  line L294 (-143.8532, -206.2865) -> (-143.8532, -207.7364)
  line L295 (-143.8532, -207.7364) -> (-143.2758, -207.7364)
  line L296 (-146.1673, -207.7364) -> (-146.1673, -203.394)
  line L297 (-146.1673, -203.394) -> (-150.3628, -203.394)
  line L298 (-150.3628, -203.394) -> (-150.3628, -207.7364)
  line L299 (-150.3628, -207.7364) -> (-146.1673, -207.7364)
  line L300 (-152.6466, -207.7364) -> (-152.6466, -203.394)
  line L301 (-152.6466, -203.394) -> (-156.9944, -203.394)
  line L302 (-156.9944, -203.394) -> (-156.9944, -207.7364)
  line L303 (-156.9944, -207.7364) -> (-152.6466, -207.7364)
  line L304 (-159.2509, -207.7364) -> (-159.2509, -203.394)
  line L305 (-159.2509, -203.394) -> (-163.616, -203.394)
  line L306 (-163.616, -203.394) -> (-163.616, -207.7364)
  line L307 (-163.616, -207.7364) -> (-159.2509, -207.7364)
  line L308 (-165.8649, -203.394) -> (-170.3485, -203.394)
  line L309 (-170.3485, -203.394) -> (-170.3485, -207.7364)
  line L310 (-170.3485, -207.7364) -> (-165.8649, -207.7364)
  line L311 (-165.8649, -207.7364) -> (-165.8649, -203.394)
  line L312 (-172.6153, -203.394) -> (-178.675, -203.394)
  line L313 (-178.675, -203.394) -> (-178.675, -207.7364)
  line L314 (-178.675, -207.7364) -> (-172.6153, -207.7364)
  line L315 (-172.6153, -207.7364) -> (-172.6153, -203.394)
  line L316 (-172.6153, -196.9098) -> (-176.5021, -196.9098)
  line L317 (-176.5021, -196.9098) -> (-178.1818, -201.1101)
  line L318 (-178.1818, -201.1101) -> (-172.6153, -201.1101)
  line L319 (-172.6153, -201.1101) -> (-172.6153, -196.9098)
  line L320 (-172.6153, -193.856) -> (-174.1802, -194.6061)
  line L321 (-174.1802, -194.6061) -> (-172.6153, -194.6061)
  line L322 (-172.6153, -194.6061) -> (-172.6153, -193.856)
  line L323 (-149.8661, -194.6061) -> (-150.3628, -194.3607)
  line L324 (-150.3628, -194.3607) -> (-150.3628, -194.6061)
  line L325 (-150.3628, -194.6061) -> (-149.8661, -194.6061)
  line L326 (-146.1673, -200.4774) -> (-147.5883, -196.9098)
  line L327 (-147.5883, -196.9098) -> (-150.3628, -196.9098)
  line L328 (-150.3628, -196.9098) -> (-150.3628, -201.1101)
  line L329 (-150.3628, -201.1101) -> (-146.1673, -201.1101)
  line L330 (-146.1673, -201.1101) -> (-146.1673, -200.4774)
  line L331 (-152.6466, -196.9098) -> (-156.9944, -196.9098)
  line L332 (-156.9944, -196.9098) -> (-156.9944, -201.1101)
  line L333 (-156.9944, -201.1101) -> (-152.6466, -201.1101)
  line L334 (-152.6466, -201.1101) -> (-152.6466, -196.9098)
  line L335 (-152.6466, -193.2326) -> (-156.9944, -191.0845)
  line L336 (-156.9944, -191.0845) -> (-156.9944, -194.6061)
  line L337 (-156.9944, -194.6061) -> (-152.6466, -194.6061)
  line L338 (-152.6466, -194.6061) -> (-152.6466, -193.2326)
  line L339 (-159.2509, -194.6061) -> (-159.2509, -189.9694)
  line L340 (-159.2509, -189.9694) -> (-161.8395, -188.6907)
  line L341 (-161.8395, -188.6907) -> (-163.616, -189.5422)
  line L342 (-163.616, -189.5422) -> (-163.616, -194.6061)
  line L343 (-163.616, -194.6061) -> (-159.2509, -194.6061)
  line L344 (-165.8649, -190.62) -> (-170.3485, -192.7692)
  line L345 (-170.3485, -192.7692) -> (-170.3485, -194.6061)
  line L346 (-170.3485, -194.6061) -> (-165.8649, -194.6061)
  line L347 (-165.8649, -194.6061) -> (-165.8649, -190.62)
  line L348 (-165.8649, -196.9098) -> (-170.3485, -196.9098)
  line L349 (-170.3485, -196.9098) -> (-170.3485, -201.1101)
  line L350 (-170.3485, -201.1101) -> (-165.8649, -201.1101)
  line L351 (-165.8649, -201.1101) -> (-165.8649, -196.9098)
  line L352 (-159.2509, -196.9098) -> (-163.616, -196.9098)
  line L353 (-163.616, -196.9098) -> (-163.616, -201.1101)
  line L354 (-163.616, -201.1101) -> (-159.2509, -201.1101)
  line L355 (-159.2509, -201.1101) -> (-159.2509, -196.9098)
  line L356 (-180.9883, -210.1559) -> (-180.9883, -210.0039)
  line L357 (-180.9883, -208.2364) -> (-180.9883, -208.1294)
  line L358 (-181.031, -208.2364) -> (-180.9883, -208.1294)
  dimension "d77" = -0.5
  dimension "d78" = -0.5
  dimension "d79" = -0.5
  dimension "d80" = -0.5
  dimension "d81" = -0.5
  dimension "d82" = -0.5
  dimension "d83" = -0.5
  dimension "d84" = -0.5
  dimension "d85" = -0.5
  dimension "d86" = -0.5
  dimension "d87" = -0.5
  dimension "d88" = -0.5
  dimension "d89" = -0.5
  dimension "d90" = -0.5
  dimension "d91" = -0.5
  dimension "d92" = -0.5
  dimension "d93" = -0.5
  dimension "d94" = -0.5
  dimension "d95" = -0.5
  dimension "d96" = -0.5
  dimension "d97" = -0.5
  dimension "d98" = -0.5
  dimension "d99" = -0.5
  dimension "d100" = -0.5
  dimension "d101" = -0.5
  dimension "d102" = -0.5
  dimension "d103" = -0.5
  dimension "d104" = -0.5
  dimension "d105" = -0.5
  dimension "d106" = -0.5
  dimension "d107" = -0.5
  dimension "d108" = -0.5
  dimension "d109" = -0.5
  dimension "d110" = -0.5
  dimension "d111" = -0.5
  dimension "d112" = -0.5
  dimension "d113" = -0.5
  dimension "d114" = -0.5
  dimension "d115" = -0.5
  dimension "d116" = -0.5
  constraint coincident L3.end L198.start
  constraint coincident L4.start L197.start
  constraint parallel L4 L197
  constraint parallel L3 L198
  constraint coincident L268 L356.start
  constraint perpendicular L96 L356
  constraint coincident L96.end L356
  constraint collinear L356 L357
extrude "Extrude3" add sketch "Sketch2" against normal blind 4.699 separate body contours L0 L1 L2 L3 L4 L5 L6 L7 L8 L9 L10 L11 L12 L13 L14 L15 L16 L17 L18 L19 L20 L21 L22 L23 L25 L26 L27 L28 L29 L30 L193 L194 L195 L196 L197 L198 | L31 L32 L33 L34 | L35 L36 L37 L38 | L39 L40 L41 L42 L43 | L44 L45 L46 L47 | L48 L49 L50 L51 | L52 L53 L54 L55 L56 | L57 L58 L59 L60 | L61 L62 L63 L64 | L65 L66 L67 L68 | L69 L70 L71 L72 | L73 L74 L75 | L76 L77 L78 L79 | L80 L81 L82 L83 | L84 L85 L86 L87 | L88 L89 L90 L91 | L92 L93 L94 L95 | L97 L98 L99 L100 | L101 L102 L103 L104 | L105 L106 L107 L108 | L109 L110 L111 L112 | L113 L114 L115 L116 | L117 L118 L119 L120 | L121 L122 L123 L124 | L125 L126 L127 L128 | L129 L130 L131 L132 | L133 L134 L135 L136 | L137 L138 L139 L140 | L141 L142 L143 L144 | L145 L146 L147 L148 | L149 L150 L151 L152 | L153 L154 L155 | L156 L157 L158 | L159 L160 L161 L162 L163 | L164 L165 L166 L167 | L168 L169 L170 L171 | L172 L173 L174 L175 | L176 L177 L178 L179 L180 | L181 L182 L183 | L184 L185 L186 L187 | L188 L189 L190 L191 L192 makes body 8
delete_body "RemoveBody1" bodies 3